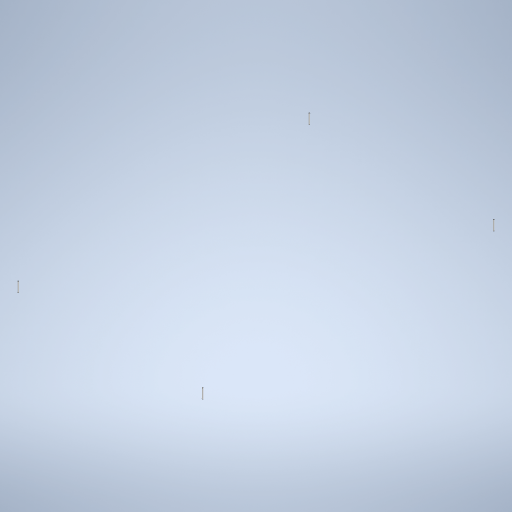
# Autodesk Inventor part: Legs
Saved by Autodesk Inventor 2024 (Build 280153000, 153)
## iProperties
Created: 2023-03-05
Part Number: Legs
Material: Generic
Document SubType Name: Modeling
Designer: sauliusd
Density: 1 g/cm^3
Appearance: Default
Author: sauliusd
Autodesk Inventor part; units mm, degrees
ref_plane "YZ Plane" through (0, 0, 0) normal (1, 0, 0) x (0, 1, 0)
ref_plane "XZ Plane" through (0, 0, 0) normal (0, 1, 0) x (-1, 0, 0)
ref_plane "XY Plane" through (0, 0, 0) normal (0, 0, 1) x (1, 0, 0)
sketch "Sketch1" plane through (0, 0, 0) normal (0, 0, 1) x (1, 0, 0)
  line L0 (-200, -150) -> (200, -150)
  line L1 (200, -150) -> (200, 150)
  line L2 (200, 150) -> (-200, 150)
  line L3 (-200, 150) -> (-200, -150)
  line L4 (-200, -150) -> (200, 150) construction
  line L5 (200, -150) -> (-200, 150) construction
  line L6 (-150, -100) -> (150, -100)
  line L7 (150, -100) -> (150, 90)
  line L8 (150, 90) -> (-150, 90)
  line L9 (-150, 90) -> (-150, -100)
  line L10 (-150, -100) -> (150, 90) construction
  line L11 (150, -100) -> (-150, 90) construction
  circle A0 centre (-150, -100) radius 0.5
  circle A1 centre (-150, 90) radius 0.5
  point P0 (0, 0)
  point P1 (0, -5)
  point P2 (0, -5)
  point P3 (0, -5)
  dimension "Length" = 400
  dimension "Width" = 300
  dimension "d3" = 145
  dimension "d4" = 300
  dimension "d5" = 190
  dimension "d7" = 200
  dimension "d8" = 1
  dimension "d9" = 1
  constraints: 24 end point, 6 midpoint, 4 parallel, 2 centre point, 2 coincident, 2 horizontal, 2 perpendicular
  measures "Length" distance of L2.end L1.end
  measures "Width" distance of L1.end L0.end
  measures "d3" distance from line of L0 point (0, -5)
  measures "d4" distance of L7.end L8.end
  measures "d5" distance of L8.end L6.start
  measures "d7" distance from line of L1 point (0, -5)
  measures "d8" diameter of A0
  measures "d9" diameter of A1
extrude "Extrusion1" add sketch "Sketch1" along normal blind 10 contours L9 A0 L6 | L6 A0 L9
extrude "Extrusion2" add sketch "Sketch1" along normal blind 10 separate body contours A1 L8 L9 | L9 L8 A1
pattern_linear "Rectangular Pattern2" count 2 spacing 300 along (1, 0, 0) of "Extrusion2" bodies 2
pattern_linear "Rectangular Pattern1" count 2 spacing 300 along (1, 0, 0) bodies 1
equation "\"d3\" = Y_Coord"
equation "\"d4\" = LX"
equation "\"d5\" = LY"
equation "\"d7\" = X_Coord"
equation "\"d19\" = LX"
equation "\"X_Coord\" = 0.5 * Length + 0.5 * Shift_X"
equation "\"Y_Coord\" = 0.5 * Width + 0.5 * Shift_Y"
equation "\"Shift_X\" = 0"
equation "\"LX\" = -2 * Margins_X + Length - Shift_X"
equation "\"LY\" = 190"
equation "\"Shift_Y\" = -10"
equation "\"Margins_X\" = 50"
body "Solid1"
body "Solid2"
